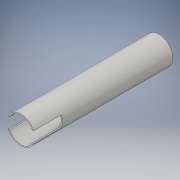
# Autodesk Inventor part: Cañón Prototipo Inicial
Saved by Autodesk Inventor 2016 SP2 (Build 200236200, 236)
## iProperties
Created: 2017-06-02
Part Number: Cañón Prototipo Inicial
Material: Tuberías de PVC
Document SubType Name: Modeling
Designer: ssant
Density: 1.4 g/cm^3
Appearance: Suave - Blanco
Author: ssant
Autodesk Inventor part; units mm, degrees
ref_plane "YZ Plane" through (0, 0, 0) normal (1, 0, 0) x (0, 1, 0)
ref_plane "XZ Plane" through (0, 0, 0) normal (0, 1, 0) x (-1, 0, 0)
ref_plane "XY Plane" through (0, 0, 0) normal (0, 0, 1) x (1, 0, 0)
sketch "Boceto1" plane through (0, 0, 0) normal (0, 0, 1) x (1, 0, 0)
  circle A0 centre (0, 0) radius 24
  dimension "d0" = 48
  constraints: 1 centre point, 1 coincident
  measures "d0" diameter of A0
extrude "Extrusión1" add sketch "Boceto1" against normal blind 250
shell "Vaciado1" thickness 2 both sides yes removed faces 2 at (5.9881, 2.1306, 0) at (5.9881, 2.1306, -250)
sketch "Boceto2" plane through (0, 0, 0) normal (1, 0, 0) x (0, 1, 0)
  line L0 (-25, -250) -> (25, -250) projected
  line L1 (-25, 0) -> (25, 0) projected
  line L2 (-25, 0) -> (25, 0) projected
  line L3 (0, 0) -> (10, 0)
  line L4 (10, 0) -> (10, -50)
  line L5 (10, -50) -> (0, -50)
  line L6 (0, -50) -> (0, 0)
  line L7 (0, 0) -> (-10, 0)
  line L8 (-10, 0) -> (-10, -50)
  line L9 (-10, -50) -> (0, -50)
  line L10 (0, -50) -> (0, 0)
  dimension "d4" = 10
  dimension "d5" = 50
  dimension "d6" = 10
  dimension "d7" = 50
  constraints: 16 end point, 4 parallel, 2 horizontal, 2 perpendicular
  measures "d4" distance of L4.end L5.end
  measures "d5" distance of L3.end L4.end
  measures "d6" distance of L9.end L8.end
  measures "d7" distance of L8.end L7.end
extrude "Extrusión2" cut sketch "Boceto2" along normal mid plane 60
